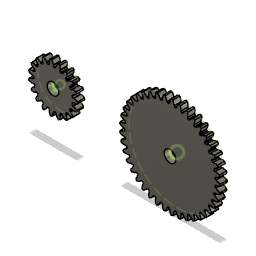
WRO Car 3D Print (Autodesk Fusion 360 design; units mm, degrees)
description: Spur Gear; Module: 1.000000; Num Teeth: 19; Pressure Angle: 20.000000; Backlash: 0.00 mm
description: Spur Gear; Module: 1.000000; Num Teeth: 41; Pressure Angle: 20.000000; Backlash: 0.00 mm
Autodesk Fusion 360 part; units mm, degrees
sketch "Sketch1" plane through (0, 0, 0) normal (0, 0, 1) x (1, 0, 0) in component "Spur Gear (19 teeth)"
  circle A0 centre (0, 0) radius 8.2492
  circle A1 centre (0, 0) radius 2.5
extrude "Extrude1" add sketch "Sketch1" along normal blind 3 makes body 1 in component "Spur Gear (19 teeth)"
sketch "Sketch2" plane through (0, 0, 0) normal (0, 0, 1) x (1, 0, 0) in component "Spur Gear (19 teeth)"
  spline S0 degree 5 poles (8.8846, -0.8697) (8.8892, -0.8701) (8.8983, -0.8709) (8.9121, -0.8717) (8.9304, -0.872) (8.9534, -0.8715) (8.9764, -0.8703) (8.9995, -0.8687) (9.0226, -0.8668) (9.0457, -0.8647) (9.0688, -0.8625) (9.0919, -0.86) (9.115, -0.8573) (9.1382, -0.8543) (9.1613, -0.8509) (9.1845, -0.8472) (9.2077, -0.8432) (9.2309, -0.839) (9.254, -0.8345) (9.2772, -0.8299) (9.3004, -0.8251) (9.3236, -0.8201) (9.3468, -0.8149) (9.37, -0.8095) (9.3932, -0.8039) (9.4164, -0.7981) (9.4395, -0.7921) (9.4627, -0.7859) (9.4859, -0.7795) (9.5091, -0.7729) (9.5322, -0.7662) (9.5554, -0.7593) (9.5786, -0.7522) (9.6017, -0.7449) (9.6249, -0.7375) (9.648, -0.7299) (9.6711, -0.7221) (9.6942, -0.7142) (9.7174, -0.7061) (9.7405, -0.6979) (9.7636, -0.6895) (9.7866, -0.6809) (9.8097, -0.6722) (9.8328, -0.6634) (9.8558, -0.6543) (9.8788, -0.6452) (9.9019, -0.6358) (9.9249, -0.6264) (9.9479, -0.6168) (9.9708, -0.607) (9.9938, -0.5971) (10.0167, -0.587) (10.0397, -0.5768) (10.0626, -0.5665) (10.0855, -0.556) (10.1084, -0.5454) (10.1312, -0.5346) (10.1541, -0.5238) (10.1769, -0.5127) (10.1997, -0.5016) (10.2225, -0.4902) (10.2453, -0.4788) (10.268, -0.4672) (10.2908, -0.4555) (10.3135, -0.4437) (10.3362, -0.4317) (10.3588, -0.4196) (10.3815, -0.4074) (10.4041, -0.395) (10.4267, -0.3825) (10.4493, -0.3699) (10.4673, -0.3597) (10.4808, -0.352) (10.4899, -0.3468) (10.4944, -0.3442) knots 0 0 0 0 0 0 0.01428571 0.02857143 0.04285714 0.05714286 0.07142857 0.08571429 0.1 0.11428571 0.12857143 0.14285714 0.15714286 0.17142857 0.18571429 0.2 0.21428571 0.22857143 0.24285714 0.25714286 0.27142857 0.28571429 0.3 0.31428571 0.32857143 0.34285714 0.35714286 0.37142857 0.38571429 0.4 0.41428571 0.42857143 0.44285714 0.45714286 0.47142857 0.48571429 0.5 0.51428571 0.52857143 0.54285714 0.55714286 0.57142857 0.58571429 0.6 0.61428571 0.62857143 0.64285714 0.65714286 0.67142857 0.68571429 0.7 0.71428571 0.72857143 0.74285714 0.75714286 0.77142857 0.78571429 0.8 0.81428571 0.82857143 0.84285714 0.85714286 0.87142857 0.88571429 0.9 0.91428571 0.92857143 0.94285714 0.95714286 0.97142857 0.98571429 1 1 1 1 1 1
  spline S1 degree 5 poles (8.8846, 0.8697) (8.8892, 0.8701) (8.8983, 0.8709) (8.9121, 0.8717) (8.9304, 0.872) (8.9534, 0.8715) (8.9764, 0.8703) (8.9995, 0.8687) (9.0226, 0.8668) (9.0457, 0.8647) (9.0688, 0.8625) (9.0919, 0.86) (9.115, 0.8573) (9.1382, 0.8543) (9.1613, 0.8509) (9.1845, 0.8472) (9.2077, 0.8432) (9.2309, 0.839) (9.254, 0.8345) (9.2772, 0.8299) (9.3004, 0.8251) (9.3236, 0.8201) (9.3468, 0.8149) (9.37, 0.8095) (9.3932, 0.8039) (9.4164, 0.7981) (9.4395, 0.7921) (9.4627, 0.7859) (9.4859, 0.7795) (9.5091, 0.7729) (9.5322, 0.7662) (9.5554, 0.7593) (9.5786, 0.7522) (9.6017, 0.7449) (9.6249, 0.7375) (9.648, 0.7299) (9.6711, 0.7221) (9.6942, 0.7142) (9.7174, 0.7061) (9.7405, 0.6979) (9.7636, 0.6895) (9.7866, 0.6809) (9.8097, 0.6722) (9.8328, 0.6634) (9.8558, 0.6543) (9.8788, 0.6452) (9.9019, 0.6358) (9.9249, 0.6264) (9.9479, 0.6168) (9.9708, 0.607) (9.9938, 0.5971) (10.0167, 0.587) (10.0397, 0.5768) (10.0626, 0.5665) (10.0855, 0.556) (10.1084, 0.5454) (10.1312, 0.5346) (10.1541, 0.5238) (10.1769, 0.5127) (10.1997, 0.5016) (10.2225, 0.4902) (10.2453, 0.4788) (10.268, 0.4672) (10.2908, 0.4555) (10.3135, 0.4437) (10.3362, 0.4317) (10.3588, 0.4196) (10.3815, 0.4074) (10.4041, 0.395) (10.4267, 0.3825) (10.4493, 0.3699) (10.4673, 0.3597) (10.4808, 0.352) (10.4899, 0.3468) (10.4944, 0.3442) knots 0 0 0 0 0 0 0.01428571 0.02857143 0.04285714 0.05714286 0.07142857 0.08571429 0.1 0.11428571 0.12857143 0.14285714 0.15714286 0.17142857 0.18571429 0.2 0.21428571 0.22857143 0.24285714 0.25714286 0.27142857 0.28571429 0.3 0.31428571 0.32857143 0.34285714 0.35714286 0.37142857 0.38571429 0.4 0.41428571 0.42857143 0.44285714 0.45714286 0.47142857 0.48571429 0.5 0.51428571 0.52857143 0.54285714 0.55714286 0.57142857 0.58571429 0.6 0.61428571 0.62857143 0.64285714 0.65714286 0.67142857 0.68571429 0.7 0.71428571 0.72857143 0.74285714 0.75714286 0.77142857 0.78571429 0.8 0.81428571 0.82857143 0.84285714 0.85714286 0.87142857 0.88571429 0.9 0.91428571 0.92857143 0.94285714 0.95714286 0.97142857 0.98571429 1 1 1 1 1 1
  arc A0 (10.4944, -0.3442) -> (10.4944, 0.3442) centre (0, 0) ccw
  line L0 (8.2, -0.8037) -> (8.8846, -0.8697)
  line L1 (8.2, 0.8037) -> (8.8846, 0.8697)
  line L2 (8.2, -0.8037) -> (8.2, 0.8037)
  point P0 (8.9976, -0.8687)
  point P1 (9.1115, -0.8577)
  point P2 (9.226, -0.8398)
  point P3 (9.3409, -0.8162)
  point P4 (9.4561, -0.7876)
  point P5 (9.5715, -0.7543)
  point P6 (9.6871, -0.7167)
  point P7 (9.8027, -0.6748)
  point P8 (9.9183, -0.629)
  point P9 (10.0339, -0.5794)
  point P10 (10.1493, -0.526)
  point P11 (10.2646, -0.469)
  point P12 (10.3796, -0.4083)
  point P13 (8.9976, 0.8687)
  point P14 (9.1115, 0.8577)
  point P15 (9.226, 0.8398)
  point P16 (9.3409, 0.8162)
  point P17 (9.4561, 0.7876)
  point P18 (9.5715, 0.7543)
  point P19 (9.6871, 0.7167)
  point P20 (9.8027, 0.6748)
  point P21 (9.9183, 0.629)
  point P22 (10.0339, 0.5794)
  point P23 (10.1493, 0.526)
  point P24 (10.2646, 0.469)
  point P25 (10.3796, 0.4083)
extrude "Extrude2" add sketch "Sketch2" along normal blind 3 bodies 1 in component "Spur Gear (19 teeth)"
fillet "Fillet1" radius 0.5 2 edges at (8.2099, -0.8046, 1.5) (8.2099, 0.8046, 1.5) on bodies 1 in component "Spur Gear (19 teeth)"
pattern_circular "C-Pattern1" count 19 over 360 about axis through (0, 0, 0) along (0, 0, 1) of "Extrude2", "Fillet1" in component "Spur Gear (19 teeth)"
sketch "Sketch3" plane through (0, 0, 0) normal (0, 0, 1) x (1, 0, 0) in component "Spur Gear (19 teeth)"
  circle A0 centre (0, 0) radius 9.5 construction
sketch "Sketch1 (2)" plane through (0, 0, 0) normal (0, 0, 1) x (1, 0, 0) in component "Spur Gear (41 teeth)"
  circle A0 centre (0, 0) radius 19.2492
  circle A1 centre (0, 0) radius 2.5
extrude "Extrude1'" add sketch "Sketch1 (2)" along normal blind 3 separate body makes body 2 in component "Spur Gear (41 teeth)"
sketch "Sketch2 (2)" plane through (0, 0, 0) normal (0, 0, 1) x (1, 0, 0) in component "Spur Gear (41 teeth)"
  spline S0 degree 5 poles (19.2364, -1.0247) (19.2429, -1.0249) (19.2559, -1.0252) (19.2754, -1.0253) (19.3014, -1.025) (19.3338, -1.0237) (19.3663, -1.0218) (19.3988, -1.0193) (19.4313, -1.0165) (19.4639, -1.0133) (19.4964, -1.0099) (19.5289, -1.0062) (19.5615, -1.0021) (19.594, -0.9978) (19.6266, -0.993) (19.6591, -0.988) (19.6916, -0.9827) (19.7241, -0.9771) (19.7567, -0.9713) (19.7892, -0.9653) (19.8217, -0.959) (19.8542, -0.9525) (19.8867, -0.9458) (19.9192, -0.9388) (19.9517, -0.9316) (19.9842, -0.9242) (20.0167, -0.9166) (20.0491, -0.9088) (20.0816, -0.9008) (20.1141, -0.8926) (20.1465, -0.8842) (20.1789, -0.8756) (20.2114, -0.8668) (20.2438, -0.8578) (20.2762, -0.8486) (20.3086, -0.8393) (20.3409, -0.8298) (20.3733, -0.8201) (20.4057, -0.8102) (20.438, -0.8001) (20.4703, -0.7899) (20.5027, -0.7795) (20.535, -0.769) (20.5673, -0.7583) (20.5995, -0.7474) (20.6318, -0.7363) (20.6641, -0.7251) (20.6963, -0.7137) (20.7285, -0.7022) (20.7607, -0.6905) (20.7929, -0.6787) (20.8251, -0.6667) (20.8572, -0.6546) (20.8894, -0.6423) (20.9215, -0.6298) (20.9536, -0.6172) (20.9857, -0.6045) (21.0178, -0.5916) (21.0498, -0.5786) (21.0819, -0.5654) (21.1139, -0.552) (21.1459, -0.5386) (21.1779, -0.525) (21.2098, -0.5112) (21.2418, -0.4973) (21.2737, -0.4833) (21.3056, -0.4691) (21.3375, -0.4548) (21.3694, -0.4404) (21.4012, -0.4258) (21.433, -0.4111) (21.4585, -0.3992) (21.4776, -0.3902) (21.4903, -0.3842) (21.4966, -0.3812) knots 0 0 0 0 0 0 0.01428571 0.02857143 0.04285714 0.05714286 0.07142857 0.08571429 0.1 0.11428571 0.12857143 0.14285714 0.15714286 0.17142857 0.18571429 0.2 0.21428571 0.22857143 0.24285714 0.25714286 0.27142857 0.28571429 0.3 0.31428571 0.32857143 0.34285714 0.35714286 0.37142857 0.38571429 0.4 0.41428571 0.42857143 0.44285714 0.45714286 0.47142857 0.48571429 0.5 0.51428571 0.52857143 0.54285714 0.55714286 0.57142857 0.58571429 0.6 0.61428571 0.62857143 0.64285714 0.65714286 0.67142857 0.68571429 0.7 0.71428571 0.72857143 0.74285714 0.75714286 0.77142857 0.78571429 0.8 0.81428571 0.82857143 0.84285714 0.85714286 0.87142857 0.88571429 0.9 0.91428571 0.92857143 0.94285714 0.95714286 0.97142857 0.98571429 1 1 1 1 1 1
  spline S1 degree 5 poles (19.2364, 1.0247) (19.2429, 1.0249) (19.2559, 1.0252) (19.2754, 1.0253) (19.3014, 1.025) (19.3338, 1.0237) (19.3663, 1.0218) (19.3988, 1.0193) (19.4313, 1.0165) (19.4639, 1.0133) (19.4964, 1.0099) (19.5289, 1.0062) (19.5615, 1.0021) (19.594, 0.9978) (19.6266, 0.993) (19.6591, 0.988) (19.6916, 0.9827) (19.7241, 0.9771) (19.7567, 0.9713) (19.7892, 0.9653) (19.8217, 0.959) (19.8542, 0.9525) (19.8867, 0.9458) (19.9192, 0.9388) (19.9517, 0.9316) (19.9842, 0.9242) (20.0167, 0.9166) (20.0491, 0.9088) (20.0816, 0.9008) (20.1141, 0.8926) (20.1465, 0.8842) (20.1789, 0.8756) (20.2114, 0.8668) (20.2438, 0.8578) (20.2762, 0.8486) (20.3086, 0.8393) (20.3409, 0.8298) (20.3733, 0.8201) (20.4057, 0.8102) (20.438, 0.8001) (20.4703, 0.7899) (20.5027, 0.7795) (20.535, 0.769) (20.5673, 0.7583) (20.5995, 0.7474) (20.6318, 0.7363) (20.6641, 0.7251) (20.6963, 0.7137) (20.7285, 0.7022) (20.7607, 0.6905) (20.7929, 0.6787) (20.8251, 0.6667) (20.8572, 0.6546) (20.8894, 0.6423) (20.9215, 0.6298) (20.9536, 0.6172) (20.9857, 0.6045) (21.0178, 0.5916) (21.0498, 0.5786) (21.0819, 0.5654) (21.1139, 0.552) (21.1459, 0.5386) (21.1779, 0.525) (21.2098, 0.5112) (21.2418, 0.4973) (21.2737, 0.4833) (21.3056, 0.4691) (21.3375, 0.4548) (21.3694, 0.4404) (21.4012, 0.4258) (21.433, 0.4111) (21.4585, 0.3992) (21.4776, 0.3902) (21.4903, 0.3842) (21.4966, 0.3812) knots 0 0 0 0 0 0 0.01428571 0.02857143 0.04285714 0.05714286 0.07142857 0.08571429 0.1 0.11428571 0.12857143 0.14285714 0.15714286 0.17142857 0.18571429 0.2 0.21428571 0.22857143 0.24285714 0.25714286 0.27142857 0.28571429 0.3 0.31428571 0.32857143 0.34285714 0.35714286 0.37142857 0.38571429 0.4 0.41428571 0.42857143 0.44285714 0.45714286 0.47142857 0.48571429 0.5 0.51428571 0.52857143 0.54285714 0.55714286 0.57142857 0.58571429 0.6 0.61428571 0.62857143 0.64285714 0.65714286 0.67142857 0.68571429 0.7 0.71428571 0.72857143 0.74285714 0.75714286 0.77142857 0.78571429 0.8 0.81428571 0.82857143 0.84285714 0.85714286 0.87142857 0.88571429 0.9 0.91428571 0.92857143 0.94285714 0.95714286 0.97142857 0.98571429 1 1 1 1 1 1
  arc A0 (21.4966, -0.3812) -> (21.4966, 0.3812) centre (0, 0) ccw
  line L0 (19.212, -1.0239) -> (19.2364, -1.0247)
  line L1 (19.212, 1.0239) -> (19.2364, 1.0247)
  line L2 (19.212, -1.0239) -> (19.212, 1.0239)
  point P0 (19.3967, -1.0194)
  point P1 (19.5575, -1.0026)
  point P2 (19.7187, -0.978)
  point P3 (19.8801, -0.9471)
  point P4 (20.0417, -0.9106)
  point P5 (20.2034, -0.8689)
  point P6 (20.3652, -0.8225)
  point P7 (20.5271, -0.7715)
  point P8 (20.6889, -0.7163)
  point P9 (20.8507, -0.657)
  point P10 (21.0124, -0.5937)
  point P11 (21.174, -0.5266)
  point P12 (21.3354, -0.4557)
  point P13 (19.3967, 1.0194)
  point P14 (19.5575, 1.0026)
  point P15 (19.7187, 0.978)
  point P16 (19.8801, 0.9471)
  point P17 (20.0417, 0.9106)
  point P18 (20.2034, 0.8689)
  point P19 (20.3652, 0.8225)
  point P20 (20.5271, 0.7715)
  point P21 (20.6889, 0.7163)
  point P22 (20.8507, 0.657)
  point P23 (21.0124, 0.5937)
  point P24 (21.174, 0.5266)
  point P25 (21.3354, 0.4557)
extrude "Extrude2'" add sketch "Sketch2 (2)" along normal blind 3 bodies 2 in component "Spur Gear (41 teeth)"
fillet "Fillet1'" radius 0.5 2 edges at (19.2219, -1.0242, 1.5) (19.2219, 1.0242, 1.5) on bodies 2 in component "Spur Gear (41 teeth)"
pattern_circular "C-Pattern1'" count 41 over 360 about axis through (0, 0, -0.0002) along (0, 0, 1) of "Extrude2'", "Fillet1'" in component "Spur Gear (41 teeth)"
sketch "Sketch3 (2)" plane through (0, 0, 0) normal (0, 0, 1) x (1, 0, 0) in component "Spur Gear (41 teeth)"
  circle A0 centre (0, 0) radius 20.5 construction
component "Spur Gear (19 teeth)" placed x (1, 0, 0) y (0, 1, 0) z (0, 0, 1) at (0, 0, 0)
component "Spur Gear (41 teeth)" placed x (1, 0, 0) y (0, 1, 0) z (0, 0, 1) at (0, 0, 0)
